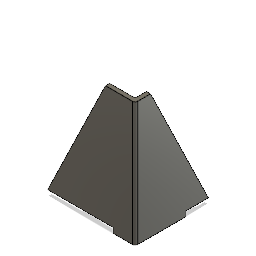
_Cage Holder.7f562d8a-6cf2-4040-be1b-836627ca3a5c (Autodesk Fusion 360 design; units mm, degrees)
Autodesk Fusion 360 part; units mm, degrees
sketch "Sketch1" plane through (0, 0, 0) normal (0, 1, 0) x (1, 0, 0)
  line L0 (151.25, 77) -> (-151.25, 77) construction
  line L1 (-151.25, 77) -> (-151.25, -77) construction
  line L2 (-151.25, -77) -> (151.25, -77) construction
  line L3 (151.25, -77) -> (151.25, 77) construction
  line L4 (151.25, 77) -> (-151.25, -77) construction
  line L5 (-151.25, 77) -> (151.25, -77) construction
  line L6 (145.665, 88.5) -> (-145.665, 88.5) construction
  line L7 (-145.665, 88.5) -> (-145.665, -88.5) construction
  line L8 (-145.665, -88.5) -> (145.665, -88.5) construction
  line L9 (145.665, -88.5) -> (145.665, 88.5) construction
  line L10 (145.665, 88.5) -> (-145.665, -88.5) construction
  line L11 (-145.665, 88.5) -> (145.665, -88.5) construction
  line L12 (145.665, 89.5) -> (-146.665, 89.5)
  line L13 (-146.665, 89.5) -> (-146.665, -89.5)
  line L14 (-146.665, -89.5) -> (145.665, -89.5)
  line L15 (146.665, -88.5) -> (146.665, 88.5)
  line L16 (-149.165, -92) -> (147.665, -92)
  line L17 (149.165, -90.5) -> (149.165, 90.5)
  line L18 (147.665, 92) -> (-149.165, 92)
  line L19 (-149.165, 92) -> (-149.165, -92)
  arc A0 (149.165, 90.5) -> (147.665, 92) centre (147.665, 90.5) ccw
  arc A1 (146.665, 88.5) -> (145.665, 89.5) centre (145.665, 88.5) ccw
  arc A2 (147.665, -92) -> (149.165, -90.5) centre (147.665, -90.5) ccw
  arc A3 (145.665, -89.5) -> (146.665, -88.5) centre (145.665, -88.5) ccw
  line L20 (97.665, 92) -> (97.665, 89.5)
  line L21 (146.665, 40.5) -> (149.165, 40.5)
  line L22 (151.25, 77) -> (136.25, 77)
  line L23 (151.25, 77) -> (151.25, 62)
  line L24 (136.25, 77) -> (136.25, 89.5)
  line L25 (151.25, 62) -> (156.25, 62)
  line L26 (156.25, 62) -> (156.25, 92)
  line L27 (156.25, 92) -> (146, 92)
  line L28 (151.25, 62) -> (149.165, 62)
  line L29 (149.165, 62) -> (146.665, 62)
  line L30 (97.665, 89.5) -> (97.665, 77)
  line L31 (97.665, 77) -> (136.25, 77)
  line L32 (136.25, 89.5) -> (136.25, 92)
  line L33 (149.1467, 77) -> (146.665, 77)
  line L34 (117.665, 89.5) -> (125.665, 89.5)
  line L35 (125.665, 89.5) -> (125.665, 65.5)
  line L36 (125.665, 65.5) -> (117.665, 65.5)
  line L37 (117.665, 65.5) -> (117.665, 89.5)
  line L38 (146.665, 68.5) -> (135.665, 68.5)
  line L39 (135.665, 68.5) -> (135.665, 60.5)
  line L40 (135.665, 60.5) -> (146.665, 60.5)
  line L41 (146.665, 60.5) -> (146.665, 68.5)
  line L42 (117.665, 89.5) -> (117.665, 92)
  line L43 (125.665, 89.5) -> (125.665, 92)
  line L44 (146.665, 60.5) -> (149.165, 60.5)
  line L45 (146.665, 68.5) -> (149.165, 68.5)
  circle A4 centre (121.665, 70.3) radius 2.8
  circle A5 centre (140.465, 64.5) radius 2.8
  circle A6 centre (121.665, 70.3) radius 1.6
  circle A7 centre (140.465, 64.5) radius 1.6
  dimension "d1" = 302.5
  dimension "d2" = 154
  dimension "d3" = 291.33
  dimension "d4" = 177
  dimension "d7" = 1.5
  dimension "d8" = 1
  dimension "d9" = 1.5
  dimension "d10" = 1
  dimension "d25" = 50
  dimension "d26" = 50
  dimension "d29" = 15
  dimension "d30" = 15
  dimension "d31" = 5
  dimension "d40" = 24
  dimension "d41" = 8
  dimension "d42" = 20
  dimension "d43" = 11
  dimension "d44" = 8
  dimension "d45" = 20
  dimension "d49" = 5.6
  dimension "d50" = 4.8
  dimension "d51" = 5.6
  dimension "d52" = 4.8
  dimension "d53" = -1.2
  dimension "d54" = -1.2
  dimension "d78" = 1
  dimension "d79" = 1
  dimension "d80" = 2.5
  dimension "d81" = 2.5
  dimension "d82" = 4
  constraint horizontal L0
  constraint perpendicular L0 L1
  constraint parallel L0 L2
  constraint parallel L1 L3
  constraint coincident L4 origin
  constraint coincident L5 origin
  constraint horizontal L6
  constraint perpendicular L6 L7
  constraint parallel L6 L8
  constraint parallel L7 L9
  constraint coincident L10 origin
  constraint coincident L11 origin
  constraint parallel L8 L16
  constraint parallel L9 L17
  constraint parallel L6 L18
  constraint parallel L7 L19
  constraint tangent L18 A0
  constraint tangent L17 A0
  constraint parallel L6 L12
  constraint parallel L7 L13
  constraint parallel L8 L14
  constraint parallel L9 L15
  constraint tangent L15 A1
  constraint tangent L12 A1
  constraint tangent L17 A2
  constraint tangent L16 A2
  constraint tangent L15 A3
  constraint tangent L14 A3
  constraint coincident L18 L20.start
  constraint coincident L12 L20.end
  constraint perpendicular L12 L20
  constraint coincident L15 L21.start
  constraint coincident L17 L21.end
  constraint perpendicular L17 L21
  constraint perpendicular L9 L22
  constraint perpendicular L22 L23
  constraint coincident L12 L24.end
  constraint perpendicular L12 L24
  constraint perpendicular L15 L25
  constraint perpendicular L18 L26
  constraint coincident L18 L27.end
  constraint perpendicular L17 L27
  constraint coincident L17 L28.end
  constraint perpendicular L17 L28
  constraint coincident L15 L29.end
  constraint perpendicular L15 L29
  constraint coincident L0 L30.end
  constraint perpendicular L0 L30
  constraint coincident L18 L32.end
  constraint perpendicular L18 L32
  constraint coincident L0 L33.start
  constraint coincident L0 L33.end
  constraint coincident L15 L33.end
  constraint horizontal L34
  constraint vertical L35
  constraint horizontal L36
  constraint vertical L37
  constraint coincident L12 L34.start
  constraint horizontal L38
  constraint vertical L39
  constraint horizontal L40
  constraint vertical L41
  constraint coincident L15 L38.start
  constraint coincident L18 L42.end
  constraint perpendicular L18 L42
  constraint coincident L18 L43.end
  constraint perpendicular L18 L43
  constraint coincident L17 L44.end
  constraint perpendicular L17 L44
  constraint coincident L17 L45.end
  constraint perpendicular L17 L45
  measures "d1" distance of L1.end L2.end
  measures "d2" distance of L0.end L1.end
  measures "d3" distance of L7.end L8.end
  measures "d4" distance of L6.end L7.end
  measures "d7" radius of A0
  measures "d8" radius of A1
  measures "d9" radius of A2
  measures "d10" radius of A3
  measures "d25" distance of A0.centre L21
  measures "d26" distance of A0.centre L20
  measures "d29" distance of L0.start L22.end
  measures "d30" distance of L0.start L23.end
  measures "d31" distance of L23.end L25.end
  measures "d40" distance of L34.start L36.end
  measures "d41" distance of L35.end L36.end
  measures "d42" distance of L20 L37
  measures "d43" distance of L38.start L38.end
  measures "d44" distance of L38.start L40.end
  measures "d45" distance of L21 L40
  measures "d49" diameter of A4
  measures "d50" distance of L36 A4.centre
  measures "d51" diameter of A5
  measures "d52" distance of L39 A5.centre
  measures "d78" distance of L6 L12
  measures "d79" distance of L9 L15
  measures "d80" distance of L12 L18
  measures "d81" distance of L15 L17
  measures "d82" distance of L35 A4.centre
extrude "Extrude5" add sketch "Sketch1" along normal blind 70 contours L12 L15 L17 L18 A0 A1 L22 L27 L32 L33 | L12 L18 L32 L43 | L12 L18 L34 L42 L43 | L15 L17 L22 L33 L45 | L12 L18 L20 L42 | L15 L17 L29 L41 L45 | L15 L17 L29 L41 L44 | L15 L17 L21 L44 makes body 1
extrude "Extrude6" add sketch "Sketch1" against normal blind 3 contours L12 L15 A1 L22 L24 | L12 L15 L17 L18 A0 A1 L22 L27 L32 L33 | L15 L17 L22 L33 L45 | L15 L17 L29 L41 L45 bodies 1
sketch "Sketch4" plane through (149.165, 0, 0) normal (1, 0, 0) x (0, 0, -1)
  line L0 (90.5, -3) -> (90.5, 70)
  line L1 (90.5, 70) -> (40.5, 70)
  line L2 (40.5, 70) -> (40.5, 0)
  line L3 (62, -3) -> (90.5, -3)
  line L4 (40.5, 0) -> (62, 0)
  line L5 (62, 0) -> (62, -3)
  line L6 (40.5, 0) -> (74.5, 70)
  dimension "d46" = 34
  constraint coincident L2.end L4.start
  constraint coincident L1 L6.end
  measures "d46" distance of L2 L6.end
sketch "Sketch5" plane through (0, 0, -92) normal (0, 0, -1) x (-1, 0, 0)
  line L0 (-97.665, 0) -> (-97.665, 70)
  line L1 (-97.665, 70) -> (-147.665, 70)
  line L2 (-147.665, 70) -> (-147.665, -3)
  line L3 (-97.665, 0) -> (-131.665, 70)
  line L4 (-136.25, 0) -> (-97.665, 0)
  line L5 (-147.665, -3) -> (-136.25, -3)
  line L6 (-136.25, -3) -> (-136.25, 0)
  dimension "d35" = 34
  constraint coincident L0.start L3.start
  constraint coincident L1 L3.end
  measures "d35" distance of L0.end L3.end
extrude "Extrude7" cut sketch "Sketch5" against normal up to surface (2.5 mm away) contours L0 L1 L3 bodies 1
extrude "Extrude8" cut sketch "Sketch4" against normal up to surface (2.5 mm away) contours L1 L2 L6 bodies 1
extrude "Extrude9" add sketch "Sketch1" along normal blind 4.5 contours L12 L31 L34 L35 L37 | L31 L35 L36 L37 | L15 L38 L39 L40 L41 | A4 | A5 | A6 | A7 bodies 1
extrude "Extrude10" cut sketch "Sketch1" along normal up to surface (4.5 mm away) contours A6 | A7 bodies 1
sketch "Sketch6" plane through (0, 4.5, 0) normal (0, 1, 0) x (-1, 0, 0)
  circle A0 centre (-121.665, -70.3) radius 1.6
  line L0 (-117.665, -65.5) -> (-125.665, -65.5)
  line L1 (-125.665, -65.5) -> (-125.665, -89.5)
  line L2 (-125.665, -89.5) -> (-117.665, -89.5)
  line L3 (-117.665, -89.5) -> (-117.665, -65.5)
  circle A1 centre (-121.665, -70.3) radius 2.8
  circle A2 centre (-140.465, -64.5) radius 2.8
extrude "Extrude11" cut sketch "Sketch6" against normal blind 2.3 contours A1 | A2 bodies 1
mirror "Mirror1" about plane through (0, 0, 0) normal (0, 0, 1) of bodies 1 makes body 2
split "Split1" by plane through (146.665, 0, 77) normal (-1, 0, 0) bodies 2 makes body 3 at (145.1257, 0, 65.0795) makes body 4 at (121.86, 23.3333, 92)
move_body "Move1" bodies 3 to x (1, 0, 0) y (0, 1, 0) z (0, 0, 1) at (0, 0, -6.5)
move_face "OffsetFaces1" offset 2 2 faces at (125.665, 1.5, 81.5) (117.665, 1.5, 73.5) on bodies 4
move_face "OffsetFaces2" offset 6.5 1 faces at (123.665, 1.5, 65.5) on bodies 4
sketch "Sketch7" plane through (0, 4.5, 0) normal (0, 1, 0) x (-1, 0, 0)
  circle A0 centre (-121.665, 70.3) radius 2.8
  line L0 (-127.665, 59) -> (-115.665, 59)
  line L1 (-115.665, 59) -> (-115.665, 89.5)
  line L2 (-115.665, 89.5) -> (-127.665, 89.5)
  line L3 (-127.665, 89.5) -> (-127.665, 59)
  circle A1 centre (-121.665, 70.3) radius 2.8
  circle A2 centre (-121.665, 63.8) radius 2.8
  circle A3 centre (-140.465, 58) radius 2.8
  line L4 (-135.665, 62) -> (-135.665, 54)
  circle A4 centre (-121.665, 70.3) radius 1.6
  circle A5 centre (-121.665, 63.8) radius 1.6
  dimension "d68" = 5.6
  dimension "d69" = 5.6
  dimension "d70" = 4.8
  dimension "d71" = 3.2
  dimension "d72" = 3.2
  constraint concentric A2 A5
  measures "d68" diameter of A1
  measures "d69" diameter of A2
  measures "d70" distance of L0 A2.centre
  measures "d71" diameter of A4
  measures "d72" diameter of A5
extrude "Extrude12" add sketch "Sketch7" against normal up to surface (4.5 mm away) contours A0 A1 | A4 bodies 4
extrude "Extrude13" cut sketch "Sketch7" against normal up to surface (4.5 mm away) contours A5 bodies 4
extrude "Extrude14" cut sketch "Sketch7" against normal blind 2.3 contours A2 bodies 4
move_face "OffsetFaces3" offset -7.5 1 faces at (148.3317, 23.3333, 51.8333) on bodies 2
combine "Combine1" operation add target body 2 tool bodies 4 3
move_face "OffsetFaces4" offset 2 2 faces at (125.665, 1.5, -81.5) (117.665, 1.5, -73.5) on bodies 1
hidden bodies 1
equation "d3 = 302.50 mm - 11.17 mm"
equation "d4 = 154 mm + 23 mm"
equation "d50 = d49 / 2 + 2 mm"
equation "d52 = d51 / 2 + 2 mm"
equation "d82 = d41 / 2"
